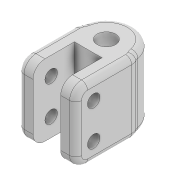
# Autodesk Inventor part: Feather_clip_acrylic
Saved by Autodesk Inventor 2022 (Build 260153000, 153)
## iProperties
Created: 2022-07-25
Part Number: Feather_clip_acrylic
Material: Generic
Document SubType Name: Modeling
Designer: dell
Density: 1 g/cm^3
Appearance: Default
Mass: 0.916016 g
Surface Area: 9.07238 cm^2
Volume: 0.916016 cm^3
Author: dell
Autodesk Inventor part; units mm, degrees
ref_plane "YZ Plane" through (0, 0, 0) normal (1, 0, 0) x (0, 1, 0)
ref_plane "XZ Plane" through (0, 0, 0) normal (0, 1, 0) x (-1, 0, 0)
ref_plane "XY Plane" through (0, 0, 0) normal (0, 0, 1) x (1, 0, 0)
sketch "Sketch1" plane through (0, 0, 0) normal (0, 1, 0) x (-1, 0, 0)
  circle A0 centre (0, 0) radius 1.55
  circle A1 centre (0, 0) radius 4.5
  dimension "d0" = 3.1
  dimension "d1" = 9
  constraints: 2 centre point, 2 coincident
  measures "d0" diameter of A0
  measures "d1" diameter of A1
extrude "Extrusion1" add sketch "Sketch1" along normal blind 12
sketch "Sketch2" plane through (0, 0, 0) normal (0, 1, 0) x (-1, 0, 0)
  line L0 (4.825, 0) -> (-4.825, 0)
  line L1 (-4.825, 0) -> (-4.825, 10)
  line L2 (-4.825, 10) -> (4.825, 10)
  line L3 (4.825, 10) -> (4.825, 0)
  line L4 (2.325, 0) -> (2.325, 10)
  line L5 (-2.325, 10) -> (-2.325, 0)
  circle A0 centre (0, 0) radius 4.5 projected
  circle A1 centre (0, 0) radius 4.5 projected
  line L6 (2.325, 3.05) -> (-2.325, 3.05)
  circle A2 centre (0, 0) radius 1.55 projected
  point P0 (-2.325, 3.8528)
  point P1 (2.325, 3.8528)
  point P2 (-4.5, 0)
  point P3 (4.5, 0)
  dimension "d4" = 4.65
  dimension "d5" = 2.325
  dimension "d6" = 2.5
  dimension "d7" = 2.5
  dimension "d8" = 10
  dimension "d25" = 1.5
  constraints: 14 end point, 6 point on line, 4 perpendicular, 2 parallel, 1 horizontal, 1 midpoint
  measures "d4" distance between parallel lines of L5 L4
  measures "d5" distance from line of L4 point (0, 0)
  measures "d6" distance between parallel lines of L4 L3
  measures "d7" distance between parallel lines of L1 L5
  measures "d8" distance from line of point (0, 0) L2
  measures "d25" distance edge to line of A2 L6
extrude "Extrusion2" add sketch "Sketch2" along normal blind 12 contours L0 A0 L4 L2 L3 | L0 L4 A0 | A0 L5 L0 | L0 L1 L2 L5 A0
extrude "Extrusion4" cut sketch "Sketch2" along normal blind 20 contours L4 L6 L5 A0 | A2 L0 | L0 A2
sketch "Sketch3" plane through (4.825, 0, 10) normal (1, 0, 0) x (0, 0, -1)
  circle A0 centre (3.05, 3.05) radius 1.05
  circle A1 centre (3.05, 8.95) radius 1.05
  line L0 (0, 0) -> (0, 12) projected
  line L1 (0, 12) -> (10, 12) projected
  line L2 (0, 0) -> (10, 0) projected
  dimension "d11" = 2.1
  dimension "d12" = 2.1
  dimension "d13" = 2
  dimension "d14" = 2
  dimension "d26" = 5.9
  dimension "d27" = 3.05
  constraints: 2 centre point
  measures "d11" diameter of A0
  measures "d12" diameter of A1
  measures "d13" distance edge to line of A1 L0
  measures "d14" distance edge to line of A0 L0
  measures "d26" distance of A0.centre A1.centre
  measures "d27" distance from line of L1 A1.centre
extrude "Extrusion3" cut sketch "Sketch3" against normal blind 11
fillet "Fillet2" radius 2 4 edges at (4.5, 6, 0) (-4.5, 6, 0) (-4.825, 6, 0) (4.825, 6, 0)
fillet "Fillet3" radius 2 4 edges at (-3.575, 12, 10) (-3.575, 0, 10) (3.575, 0, 10) (3.575, 12, 10)
fillet "Fillet4" radius 1 16 edges at (0, 12, -4.5) (4.4886, 12, -0.6014) (-4.4886, 12, -0.6014) (-4.825, 12, 4.2892) (-4.825, 11.4142, 9.4142) (-4.825, 6, 10) (-4.825, 0.5858, 9.4142) (-4.825, 0, 4.2892) (4.4886, 0, -0.6014) (-4.4886, 0, -0.6014) (0, 0, -4.5) (4.825, 0, 4.2892) (4.825, 0.5858, 9.4142) (4.825, 6, 10) (4.825, 11.4142, 9.4142) (4.825, 12, 4.2892)
equation "\"d5\" = 0.5 * d4"
body "Solid1"
